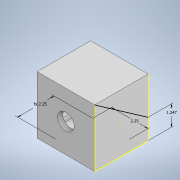
# Autodesk Inventor part: changedirection
Saved by Autodesk Inventor 2022.2 (Build 262287030, 287C)
## iProperties
Created: 2022-03-03
Part Number: changedirection
Material: Generic
Document SubType Name: Modeling
Designer: Tapendra
Density: 1 g/cm^3
Appearance: Default
Author: Tapendra
Autodesk Inventor part; units mm, degrees
ref_plane "YZ Plane" through (0, 0, 0) normal (1, 0, 0) x (0, 1, 0)
ref_plane "XZ Plane" through (0, 0, 0) normal (0, 1, 0) x (-1, 0, 0)
ref_plane "XY Plane" through (0, 0, 0) normal (0, 0, 1) x (1, 0, 0)
sketch "Sketch1" plane through (0, 0, 0) normal (0, 0, 1) x (1, 0, 0)
  line L0 (-17.78, 17.78) -> (17.78, 17.78)
  line L1 (17.78, 17.78) -> (17.78, -17.78)
  line L2 (17.78, -17.78) -> (-17.78, -17.78)
  line L3 (-17.78, -17.78) -> (-17.78, 17.78)
  line L4 (-17.78, 17.78) -> (17.78, -17.78) construction
  line L5 (17.78, 17.78) -> (-17.78, -17.78) construction
  point P0 (0, 0)
  dimension "d0" = 35.56
  dimension "d1" = 35.56
  constraints: 12 end point, 2 midpoint, 2 parallel, 1 horizontal, 1 perpendicular
  measures "d0" distance of L0.start L0.end
  measures "d1" distance of L0.end L1.end
extrude "Extrusion1" add sketch "Sketch1" along normal mid plane 33
sketch "Sketch2" plane through (-17.78, -17.78, 16.5) normal (0, -1, 0) x (1, 0, 0)
  line L0 (29.03, -27.75) -> (6.53, -27.75)
  line L1 (6.53, -27.75) -> (6.53, -5.25)
  line L2 (6.53, -5.25) -> (29.03, -5.25)
  line L3 (29.03, -5.25) -> (29.03, -27.75)
  line L4 (29.03, -27.75) -> (6.53, -5.25) construction
  line L5 (6.53, -27.75) -> (29.03, -5.25) construction
  point P0 (17.78, -16.5)
  dimension "d4" = 22.5
  dimension "d5" = 22.5
  constraints: 12 end point, 2 midpoint, 2 parallel, 1 horizontal, 1 perpendicular
  measures "d4" distance of L0.start L0.end
  measures "d5" distance of L0.end L1.end
sketch "Sketch3" plane through (17.78, -17.78, 16.5) normal (1, 0, 0) x (0, 0, -1)
  line L0 (0, 0) -> (0, 35.56) projected
  line L1 (0, 35.56) -> (33, 12.4725)
  line L2 (33, 35.56) -> (33, 0) projected
  line L3 (33, 0) -> (0, 0) projected
  point P0 (16.5, 17.78)
  dimension "d6" = 12.4725
  constraints: 2 end point, 1 point on line
  measures "d6" distance from line of L3 L1.end
sketch "Sketch4" plane through (0, 0, -16.5) normal (0, 0, -1) x (-1, 0, 0)
  line L0 (15.78, 15.78) -> (-15.78, 15.78)
  line L1 (-15.78, 15.78) -> (-15.78, -15.78)
  line L2 (-15.78, -15.78) -> (15.78, -15.78)
  line L3 (15.78, -15.78) -> (15.78, 15.78)
  line L4 (15.78, 15.78) -> (-15.78, -15.78) construction
  line L5 (-15.78, 15.78) -> (15.78, -15.78) construction
  point P0 (0, 0)
  dimension "d7" = 31.56
  dimension "d8" = 31.56
  constraints: 12 end point, 2 midpoint, 2 parallel, 1 horizontal, 1 perpendicular
  measures "d7" distance of L2.end L0.start
  measures "d8" distance of L1.end L2.end
extrude "Extrusion2" cut sketch "Sketch4" against normal blind 30
sketch "Sketch5" plane through (0, 0, 16.5) normal (0, 0, 1) x (1, 0, 0)
  circle A0 centre (0, 0) radius 5.06
  dimension "d11" = 10.12
  constraints: 1 centre point, 1 coincident
  measures "d11" diameter of A0
extrude "Extrusion3" cut sketch "Sketch5" against normal through all
sketch "Sketch6" plane through (-17.78, -17.78, 16.5) normal (-1, 0, 0) x (0, 0, 1)
  circle A0 centre (-15.24, 6.6) radius 1.7015
  line L0 (0, 0) -> (-33, 0) projected
  line L1 (-33, 0) -> (-33, 35.56) projected
  line L2 (0, 35.56) -> (0, 0) projected
  point P0 (-16.5, 17.78)
  dimension "d14" = 6.6
  dimension "d18" = 15.24
  constraints: 1 centre point
  measures "d14" distance from line of L0 A0.centre
  measures "d18" distance from line of L2 A0.centre
extrude "Extrusion4" cut sketch "Sketch6" against normal blind 2
equation "\"d1\" = d0"
equation "\"d5\" = d4"
equation "\"d8\" = d7"
body "Solid1"
